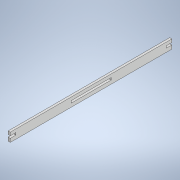
# Autodesk Inventor part: insert spacer - v2
Saved by Autodesk Inventor 2022 (Build 260153000, 153)
## iProperties
Created: 2022-07-08
Part Number: insert spacer - v2
Material: Generic
Document SubType Name: Modeling
Designer: Caleb
Density: 1 g/cm^3
Appearance: Default
Author: Caleb
Autodesk Inventor part; units mm, degrees
ref_plane "YZ Plane" through (0, 0, 0) normal (1, 0, 0) x (0, 1, 0)
ref_plane "XZ Plane" through (0, 0, 0) normal (0, 1, 0) x (-1, 0, 0)
ref_plane "XY Plane" through (0, 0, 0) normal (0, 0, 1) x (1, 0, 0)
sketch "Sketch1" plane through (0, 0, 0) normal (1, 0, 0) x (0, 1, 0)
  line L0 (-1, -18.275) -> (1, -18.275)
  line L1 (1, -18.275) -> (1, 18.275)
  line L2 (1, 18.275) -> (-1, 18.275)
  line L3 (-1, 18.275) -> (-1, -18.275)
  line L4 (-1, -18.275) -> (1, 18.275) construction
  line L5 (1, -18.275) -> (-1, 18.275) construction
  point P0 (0, 0)
  dimension "d0" = 2
  dimension "d1" = 36.55
  constraints: 12 end point, 2 midpoint, 2 parallel, 1 horizontal, 1 perpendicular
  measures "d0" distance of L1.end L2.end
  measures "d1" distance of L0.end L1.end
extrude "Extrusion1" add sketch "Sketch1" along normal blind 0.5
sketch "Sketch2" plane through (0.5, 0, 0) normal (1, 0, 0) x (0, 0, -1)
  line L0 (-18.275, 1) -> (-18.275, -1) projected
  line L1 (-18.275, 0.3) -> (-17.025, 0.3)
  line L2 (-17.025, 0.3) -> (-17.025, -0.2)
  line L3 (-17.025, -0.2) -> (-18.275, -0.2)
  line L4 (-18.275, -0.2) -> (-18.275, 0.3)
  line L5 (0, 1.1867) -> (0, -1.275)
  line L6 (18.275, 1) -> (18.275, -1)
  line L7 (18.275, 0.3) -> (17.025, 0.3)
  line L8 (17.025, 0.3) -> (17.025, -0.2)
  line L9 (17.025, -0.2) -> (18.275, -0.2)
  line L10 (18.275, -0.2) -> (18.275, 0.3)
  line L11 (18.275, 1) -> (-18.275, 1) projected
  point P0 (0, 0)
  dimension "d4" = 0.5
  dimension "d6" = 1.25
  dimension "d9" = 0.7
  constraints: 20 end point, 6 symmetric about line, 2 parallel, 2 point on line, 1 horizontal, 1 perpendicular, 1 vertical
  measures "d4" distance of L1.end L2.end
  measures "d6" distance of L1.start L1.end
  measures "d9" distance between parallel lines of L11 L1
extrude "Extrusion2" cut sketch "Sketch2" against normal blind 0.6
sketch "Sketch3" plane through (0.5, 0, 0) normal (1, 0, 0) x (0, 0, -1)
  line L0 (-18.275, -1) -> (18.275, -1) projected
  line L1 (-0.75, -1) -> (0, -0.25)
  line L2 (0, -0.25) -> (0.75, -1)
  point P0 (0, 0)
  dimension "d10" = 45
  dimension "d11" = 45
  dimension "d12" = 1.5
  constraints: 4 end point, 2 point on line, 1 vertical alignment
  measures "d10" angle of L0 L1
  measures "d11" angle of L0 L2
  measures "d12" distance of L1.start L2.end
extrude "Extrusion3" [suppressed]
sketch "Sketch4" plane through (0.5, 0, 0) normal (1, 0, 0) x (0, 0, -1)
  line L0 (-4.525, -0.2) -> (4.525, -0.2)
  line L1 (4.525, -0.2) -> (4.525, 0.3)
  line L2 (4.525, 0.3) -> (-4.525, 0.3)
  line L3 (-4.525, 0.3) -> (-4.525, -0.2)
  line L4 (-17.025, 0.3) -> (-17.025, -0.2) projected
  line L5 (18.275, 1) -> (-18.275, 1) projected
  point P0 (0, 0)
  dimension "d15" = 0.5
  dimension "d16" = 0.5
  dimension "d17" = 9.05
  dimension "d18" = 4.525
  dimension "d19" = 0.7
  constraints: 8 end point, 2 parallel, 1 horizontal, 1 perpendicular
  measures "d15" distance between parallel lines of L2 L0
  measures "d16" distance of L4.start L4.end
  measures "d17" distance of L1.end L2.end
  measures "d18" distance from line of L3 point (0, 0)
  measures "d19" distance between parallel lines of L5 L2
extrude "Extrusion4" cut sketch "Sketch4" against normal blind 10
equation "\"d11\" = d10"
equation "\"d15\" = d16"
equation "\"d18\" = 0.5 * d17"
body "Solid1"
